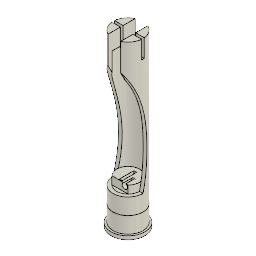
Electronic Case v1 (Autodesk Fusion 360 design; units mm, degrees)
Autodesk Fusion 360 part; units mm, degrees
note: some values were not read from the file. Chosen so that the rebuilt part matches the saved one: which face or edge a step refers to. Set by a fixed rule: which sketch regions a step uses.
sketch "Bottom" plane through (0, 0, 0) normal (0, 0, 1) x (1, 0, 0) in component "Board Case"
  circle A0 centre (0, 0) radius 6.4
  circle A1 centre (0, 0) radius 8.4
  line L0 (-8.4, 0) -> (8.4, 0) construction
  line L1 (0, 0) -> (0, 8.4) construction
  line L2 (0, 0) -> (0, -4.525) construction
  line L3 (-4.526, -4.525) -> (4.526, -4.525)
  dimension "d1" = 12.8
  dimension "d2" = 16.8
  dimension "d3" = 4.525
  measures "d1" diameter of A0
  measures "d2" diameter of A1
  measures "d3" distance of A0.centre L2.end
extrude "Extrude1" add sketch "Bottom" along normal blind 9 contours A0 L3 | A1 picked at (1.2786, -4.7244) makes body 1 in component "Board Case"
extrude "Extrude4" add sketch "Bottom" along normal blind 63 from surface at 9 bodies 1 in component "Board Case"
sketch "Top" plane through (0, 0, 72) normal (0, 0, 1) x (-1, 0, 0) in component "Board Case"
  arc A0 (4.526, 4.525) -> (-4.526, 4.525) centre (0, 0) ccw
  line L0 (-8.3665, -0.75) -> (8.3665, -0.75)
  circle A1 centre (0, 0) radius 6.4
  line L1 (8.3665, 0.75) -> (-8.3665, 0.75)
  circle A2 centre (0, 0) radius 8.4
  line L2 (-3.5, 7.6361) -> (-3.5, -7.6361)
  line L3 (3.5, -7.6361) -> (3.5, 7.6361)
  circle A3 centre (0, 0) radius 6.4
  circle A4 centre (0, 0) radius 8.4
  dimension "d6" = 16.7329
  dimension "d8" = 15.2722
  measures "d6" distance of L1.start L1.end
  measures "d8" distance of L3.start L3.end
extrude "Extrude5" add sketch "Top" along normal blind 2 contours A0 A1 L1 L3 A3 | A0 A1 L1 A2 L3 A3 A4 | L0 A1 L1 A2 A3 A4 | L0 A1 L1 L3 A3 | A0 A1 L1 L2 A3 | A0 A1 L1 A2 L2 A3 A4 | L0 A1 L1 L2 A3 | L0 A1 L3 A3 | L0 A1 A2 L3 A3 A4 | L0 A1 L1 A2 A3 A4 | L0 A1 L2 A3 | L0 A1 A2 L2 A3 A4 bodies 1 in component "Board Case"
extrude "Extrude6" add sketch "Top" along normal blind 12 contours A0 A1 L1 L3 A3 | A0 A1 L1 A2 L3 A3 A4 | A0 A1 L1 L2 A3 | A0 A1 L1 A2 L2 A3 A4 | L0 A1 L3 A3 | L0 A1 A2 L3 A3 A4 | L0 A1 L2 A3 | L0 A1 A2 L2 A3 A4 bodies 1 in component "Board Case"
sketch "Profile" plane through (0, 0, 0) normal (1, 0, 0) x (0, 1, 0) in component "Board Case"
  arc A0 (-0.0009, 8.9964) -> (-9, 71) centre (-77.9729, 29.3346) ccw
  line L0 (-9, 71) -> (-9.0491, 9.0036)
  line L1 (-9.0491, 9.0036) -> (-0.0009, 8.9964)
  point P0 (-4.525, 9)
  point P1 (-4.525, 9)
extrude "Extrude7" cut sketch "Profile" along normal mid plane 18 bodies 1 in component "Board Case"
extrude "Extrude8" cut 1 faces at (2.5666, -7.2759, 72) along direction (0, 0, -1) blind 10 on bodies 1 bodies 1 in component "Board Case"
fillet "Fillet1" radius 2.75 2 edges at (-3.5, 0, 72) (3.5, 0, 72) on bodies 1 in component "Board Case"
sketch "Profile (2)" plane through (0, 0, 0) normal (1, 0, 0) x (0, 0, -1) in component "Interior Sensors"
  line L0 (0, 0) -> (9.5, 0)
  line L1 (8.4, 2) -> (8.4, 11)
  line L2 (8.4, 11) -> (6.4, 11)
  line L3 (6.4, 24.4) -> (0, 24.4)
  line L4 (0, 24.4) -> (0, 0)
  line L5 (9.5, 0) -> (9.5, 2)
  line L6 (9.5, 2) -> (8.4, 2)
  line L7 (6.4, 24.4) -> (6.4, 11)
  dimension "r_exterrior" = 9.5
  dimension "r_interior" = 6.4
  dimension "height_bottom" = 2
  dimension "d175" = 2
  dimension "height1" = 13.4
  dimension "d237" = 9
  measures "r_exterrior" distance of L0.start L0.end
  measures "r_interior" distance of L3.start L3.end
  measures "height_bottom" distance of L0.end L5.end
  measures "d175" distance of L1.end L2.end
  measures "height1" distance of L3.start L2.end
  measures "d237" distance of L1.end L1.start
revolve "Revolve1" add sketch "Profile (2)" angle 360 about axis through (0, 24.4, 0) along (0, -1, 0) separate body makes body 2 in component "Interior Sensors"
sketch "Bottom (2)" plane through (0, 0, 0) normal (0, 1, 0) x (1, 0, 0) in component "Interior Sensors"
  line L0 (4.05, 0.8) -> (3.5217, 0.8)
  line L1 (3.5217, 0.8) -> (3.5217, 2.8)
  line L2 (-3.5217, 2.8) -> (-3.5217, 0.8)
  line L3 (-4.05, 0) -> (4.05, 0) construction
  line L4 (4.05, 0.8) -> (4.05, 0)
  line L5 (-4.05, 0.8) -> (-4.05, 0)
  arc A0 (3.5217, 2.8) -> (-3.5217, 2.8) centre (0, 4.8) ccw
  line L6 (0, 0) -> (0, 8.85) construction
  line L7 (3.5217, 0.8) -> (0, 0.8)
  line L8 (3.5217, 2.8) -> (-3.5217, 2.8) construction
  line L9 (0, 0.8) -> (-4.05, 0.8)
  line L10 (4.05, -0.8) -> (4.05, 0)
  line L11 (3.5217, -0.8) -> (3.5217, -2.8)
  line L12 (4.05, -0.8) -> (3.5217, -0.8)
  line L13 (3.5217, -0.8) -> (0, -0.8)
  line L14 (0, -0.8) -> (-4.05, -0.8)
  line L15 (-3.5217, -2.8) -> (-3.5217, -0.8)
  line L16 (-4.05, -0.8) -> (-4.05, 0)
  arc A1 (-3.5217, -2.8) -> (3.5217, -2.8) centre (0, -4.8) ccw
  dimension "diam_sensor" = 8.1
  dimension "width_joint" = 2
  dimension "d230" = 2
  dimension "d232" = 2
  dimension "width_sensor" = 0.8
  dimension "long_sensor" = 4.05
  dimension "d235" = 4.05
  measures "diam_sensor" diameter of A0
  measures "width_joint" distance of L0.end L1.end
  measures "d230" distance of L2.start L2.end
  measures "d232" distance of A0.centre L8
  measures "width_sensor" distance of L0.start L3.end
  measures "long_sensor" distance of L3.end L6.start
  measures "d235" distance of L3.start L6.start
extrude "Extrude41" cut sketch "Bottom (2)" along normal blind 26 contours L0 L4 L5 L7 L9 L10 L12 L13 L14 L16 bodies 2 in component "Interior Sensors"
extrude "Extrude45" cut sketch "Bottom (2)" along normal blind 0.9 contours L11 L13 L14 L15 A1 bodies 2 in component "Interior Sensors"
extrude "Extrude54" cut sketch "Bottom (2)" along normal blind 0.7 contours L1 L2 A0 L7 L9 bodies 2 in component "Interior Sensors"
sketch "Top (2)" plane through (0, 24.4, 0) normal (0, 1, 0) x (-1, 0, 0) in component "Interior Sensors"
  line L0 (-4.5255, -4.5255) -> (4.5255, -4.5255)
  line L1 (4.5255, -4.5255) -> (4.5255, 4.5255)
  line L2 (4.5255, 4.5255) -> (-4.5255, 4.5255)
  line L3 (-4.5255, 4.5255) -> (-4.5255, -4.5255)
  line L4 (-4.5255, -4.5255) -> (4.5255, 4.5255) construction
  line L5 (4.5255, -4.5255) -> (-4.5255, 4.5255) construction
  line L6 (4.05, -0.8) -> (-4.05, -0.8)
  line L7 (-4.05, -0.8) -> (-4.05, 0.8)
  line L8 (-4.05, 0.8) -> (4.05, 0.8)
  line L9 (4.05, 0.8) -> (4.05, -0.8)
  circle A0 centre (0, 0) radius 6.4
extrude "Extrude46" cut sketch "Top (2)" against normal blind 13.4 contours L3 A0 bodies 2 in component "Interior Sensors"
sketch "Side" plane through (4.5255, 0, 0) normal (1, 0, 0) x (0, 0, -1) in component "Interior Sensors"
  line L0 (4.5255, 24.4) -> (-4.5255, 24.4)
  line L1 (-4.5255, 24.4) -> (-4.5255, 11)
  line L2 (-4.5255, 11) -> (4.5255, 11)
  line L3 (4.5255, 11) -> (4.5255, 24.4)
  circle A0 centre (2.7627, 23) radius 1.5
  dimension "d208" = 3
  measures "d208" diameter of A0
extrude "Extrude51" cut sketch "Side" against normal blind 5 contours L0 A0 | L0 A0 bodies 2 in component "Interior Sensors"
component "Board Case" placed x (1, 0, 0) y (0, 1, 0) z (0, 0, 1) at (0, 0, 0)
component "Interior Sensors" placed x (0, -1, 0) y (0, 0, 1) z (-1, 0, 0) at (0, 0, -11)
equation "d151 = height_total"
equation "height_sensor = height_sensor1"
equation "d175 = height_bottom"
equation "d177 = -height1"
equation "d230 = width_joint"
equation "d232 = width_joint"
equation "d235 = long_sensor"
equation "height_total = 26.00 mm"
equation "height_sensor1 = 0.9 mm"
equation "height_sensor2 = 0.7 mm"
equation "d245 = height_sensor2"
named bodies: "Board", "Interior"
